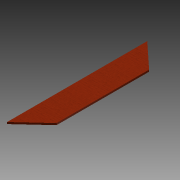
# Autodesk Inventor part: Ramp - End - Trapezoid Plywood 375
Saved by Autodesk Inventor 2015 (Build 190159000, 159)
## iProperties
Created: 2015-01-21
Part Number: Ramp - End - Trapezoid Plywood 375
Material: Wood (Oak)
Document SubType Name: Modeling
Designer: peters
Density: 0.76 g/cm^3
Appearance: White Oak - Natural Medium Gloss
Author: peters
Autodesk Inventor part; units mm, degrees
ref_plane "YZ Plane" through (0, 0, 0) normal (1, 0, 0) x (0, 1, 0)
ref_plane "XZ Plane" through (0, 0, 0) normal (0, 1, 0) x (-1, 0, 0)
ref_plane "XY Plane" through (0, 0, 0) normal (0, 0, 1) x (1, 0, 0)
sketch "Sketch1" plane through (0, 0, 0) normal (0, 1, 0) x (-1, 0, 0)
  line L0 (0, 0) -> (0, -495.3)
  line L1 (0, -495.3) -> (137.16, -622.3)
  line L2 (137.16, -622.3) -> (137.16, 127)
  line L3 (137.16, 127) -> (0, 0)
  dimension "d0" = 495.3
  dimension "d1" = 749.3
  dimension "d2" = 137.16
  constraints: 8 end point, 1 equal length, 1 parallel, 1 vertical
  measures "d0" distance of L0.start L0.end
  measures "d1" distance of L1.end L2.end
  measures "d2" distance between parallel lines of L0 L2
extrude "Extrusion1" add sketch "Sketch1" along normal blind 9.525
body "Solid1"
